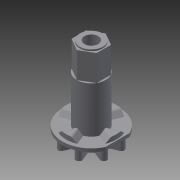
# Autodesk Inventor part: Picaporte
Saved by Autodesk Inventor 2014 (Build 180170000, 170)
## iProperties
Created: 2015-02-11
Part Number: Picaporte
Material: Generic
Document SubType Name: Modeling
Designer: Rubén
Density: 1 g/cm^3
Appearance: Default
Author: Rubén
Autodesk Inventor part; units mm, degrees
ref_plane "YZ Plane" through (0, 0, 0) normal (1, 0, 0) x (0, 1, 0)
ref_plane "XZ Plane" through (0, 0, 0) normal (0, 1, 0) x (-1, 0, 0)
ref_plane "XY Plane" through (0, 0, 0) normal (0, 0, 1) x (1, 0, 0)
sketch "Sketch1" plane through (0, 0, 0) normal (0, 1, 0) x (-1, 0, 0)
  arc A0 (-9.1, -4.1461) -> (-9.1, 4.1461) centre (0, 0) ccw
  line L0 (-9.1, 4.1461) -> (-9.1, -4.1461)
  dimension "d4" = 20
  dimension "d5" = 19.1
  constraints: 2 end point, 2 point on circle, 1 centre point, 1 coincident, 1 vertical
  measures "d4" diameter of A0
extrude "Extrusion1" add sketch "Sketch1" along normal blind 1.12
sketch "Sketch3" plane through (0, 1.12, 0) normal (0, 1, 0) x (1, 0, 0)
  arc A0 (9.1, 4.1461) -> (9.1, -4.1461) centre (0, 0) ccw projected
  circle A1 centre (0, 0) radius 5
  dimension "d14" = 10
  constraints: 1 centre point, 1 coincident
  measures "d14" diameter of A1
extrude "Extrusion3" add sketch "Sketch3" along normal blind 16
sketch "Sketch4" plane through (0, 17.12, 0) normal (0, 1, 0) x (1, 0, 0)
  circle A0 centre (0, 0) radius 5 projected
  line L0 (0, 5) -> (4.3301, 2.5)
  line L1 (4.3301, 2.5) -> (4.3301, -2.5)
  line L2 (4.3301, -2.5) -> (0, -5)
  line L3 (0, -5) -> (-4.3301, -2.5)
  line L4 (-4.3301, -2.5) -> (-4.3301, 2.5)
  line L5 (-4.3301, 2.5) -> (0, 5)
  constraints: 12 end point, 1 coincident, 1 vertical alignment, 14 other
extrude "Extrusion4" add sketch "Sketch4" along normal blind 9 contours L1 L2 L3 L4 L5 L0
sketch "Sketch5" plane through (0, 26.12, 0) normal (0, 1, 0) x (1, 0, 0)
  circle A0 centre (0, 0) radius 4
  dimension "d19" = 8
  constraints: 1 centre point, 1 coincident
  measures "d19" diameter of A0
extrude "Extrusion5" add sketch "Sketch5" along normal blind 0.5
sketch "Sketch6" plane through (0, 26.62, 0) normal (0, 1, 0) x (1, 0, 0)
  circle A0 centre (0, 0) radius 4 projected
hole "Hole1" at (0, 26.62, 0) direction (0, -1, 0) diameter 4.8 end through all
sketch "Sketch7" plane through (0, 1.12, 0) normal (0, 1, 0) x (1, 0, 0)
  circle A0 centre (0, 0) radius 5 projected
  arc A1 (9.1, 4.1461) -> (9.1, -4.1461) centre (0, 0) ccw projected
  arc A2 (3.25, 8.124) -> (-3.25, 8.124) centre (0, 0) ccw
  line L0 (0, 11.889) -> (0, 0) construction
  line L1 (-3.25, 8.124) -> (-1.8571, 4.6423)
  line L2 (3.25, 8.124) -> (1.8571, 4.6423)
  arc A3 (1.8571, 4.6423) -> (-1.8571, 4.6423) centre (0, 0) ccw
  arc A4 (-8.124, 3.25) -> (-8.124, -3.25) centre (0, 0) ccw
  line L3 (-8.124, -3.25) -> (-4.6423, -1.8571)
  line L4 (-8.124, 3.25) -> (-4.6423, 1.8571)
  arc A5 (-4.6423, 1.8571) -> (-4.6423, -1.8571) centre (0, 0) ccw
  arc A6 (-3.25, -8.124) -> (3.25, -8.124) centre (0, 0) ccw
  line L5 (3.25, -8.124) -> (1.8571, -4.6423)
  line L6 (-3.25, -8.124) -> (-1.8571, -4.6423)
  arc A7 (-1.8571, -4.6423) -> (1.8571, -4.6423) centre (0, 0) ccw
  arc A8 (8.124, -3.25) -> (8.124, 3.25) centre (0, 0) ccw
  line L7 (8.124, 3.25) -> (4.6423, 1.8571)
  line L8 (8.124, -3.25) -> (4.6423, -1.8571)
  arc A9 (4.6423, -1.8571) -> (4.6423, 1.8571) centre (0, 0) ccw
  dimension "d32" = 17.5
  dimension "d34" = 1.8571
  dimension "d35" = 3.25
  dimension "d36" = 4.6423
  dimension "d39" = 360
  constraints: 18 end point, 16 point on circle, 8 centre point, 2 symmetric about line, 1 coincident, 43 other
  measures "d32" diameter of A2
  measures "d34" distance from line of L0 L1.end
  measures "d35" distance from line of L0 L1.start
  measures "d36" vertical distance of point (0, 0) L1.end
extrude "Extrusion6" add sketch "Sketch7" along normal blind 1.6 contours A0 L7 A8 L8 | A0 L1 A2 L2 | L5 A6 L6 A0 | A0 L3 A4 L4
chamfer "Chamfer2" distance 1.6 angle 45 8 edges at (-2.5536, 2.72, -6.3832) (2.5536, 2.72, -6.3832) (-6.3832, 2.72, -2.5536) (-6.3832, 2.72, 2.5536) (-2.5536, 2.72, 6.3832) (2.5536, 2.72, 6.3832) (6.3832, 2.72, 2.5536) (6.3832, 2.72, -2.5536)
fillet "Fillet1" radius 1 8 edges at (6.7869, 2.72, -0.9919) (6.7869, 2.72, 0.9919) (0.9919, 2.72, 6.7869) (-0.9919, 2.72, 6.7869) (-6.7869, 2.72, 0.9919) (-6.7869, 2.72, -0.9919) (-0.9919, 2.72, -6.7869) (0.9919, 2.72, -6.7869)
sketch "Sketch8" plane through (0, 0, 0) normal (0, -1, 0) x (1, 0, 0)
  circle A0 centre (0, 0) radius 2.4 projected
  arc A1 (9.1, 4.1461) -> (9.1, -4.1461) centre (0, 0) ccw projected
  line L0 (0, 0) -> (9.2388, 3.8268) construction
  line L1 (0, 0) -> (10, 0) construction
  line L2 (3.9195, 2.7708) -> (6.9854, 4.0408)
  line L3 (8.292, 3.4996) -> (8.3149, 3.4442)
  arc A2 (8.292, 3.4996) -> (6.9854, 4.0408) centre (7.3681, 3.1169) ccw
  line L4 (4.7308, 0.8122) -> (7.7967, 2.0822)
  line L5 (8.3379, 3.3887) -> (8.3149, 3.4442)
  arc A3 (7.7967, 2.0822) -> (8.3379, 3.3887) centre (7.414, 3.006) ccw
  line L6 (0.8122, 4.7308) -> (2.0822, 7.7967)
  line L7 (3.3887, 8.3379) -> (3.4442, 8.3149)
  arc A4 (3.3887, 8.3379) -> (2.0822, 7.7967) centre (3.006, 7.414) ccw
  line L8 (2.7708, 3.9195) -> (4.0408, 6.9854)
  arc A5 (4.0408, 6.9854) -> (3.4996, 8.292) centre (3.1169, 7.3681) ccw
  line L9 (3.4996, 8.292) -> (3.4442, 8.3149)
  line L10 (-2.7708, 3.9195) -> (-4.0408, 6.9854)
  line L11 (-3.4996, 8.292) -> (-3.4442, 8.3149)
  arc A6 (-3.4996, 8.292) -> (-4.0408, 6.9854) centre (-3.1169, 7.3681) ccw
  line L12 (-0.8122, 4.7308) -> (-2.0822, 7.7967)
  arc A7 (-2.0822, 7.7967) -> (-3.3887, 8.3379) centre (-3.006, 7.414) ccw
  line L13 (-3.3887, 8.3379) -> (-3.4442, 8.3149)
  line L14 (-4.7308, 0.8122) -> (-7.7967, 2.0822)
  line L15 (-8.3379, 3.3887) -> (-8.3149, 3.4442)
  arc A8 (-8.3379, 3.3887) -> (-7.7967, 2.0822) centre (-7.414, 3.006) ccw
  line L16 (-3.9195, 2.7708) -> (-6.9854, 4.0408)
  arc A9 (-6.9854, 4.0408) -> (-8.292, 3.4996) centre (-7.3681, 3.1169) ccw
  line L17 (-8.292, 3.4996) -> (-8.3149, 3.4442)
  line L18 (-3.9195, -2.7708) -> (-6.9854, -4.0408)
  line L19 (-8.292, -3.4996) -> (-8.3149, -3.4442)
  arc A10 (-8.292, -3.4996) -> (-6.9854, -4.0408) centre (-7.3681, -3.1169) ccw
  line L20 (-4.7308, -0.8122) -> (-7.7967, -2.0822)
  arc A11 (-7.7967, -2.0822) -> (-8.3379, -3.3887) centre (-7.414, -3.006) ccw
  line L21 (-8.3379, -3.3887) -> (-8.3149, -3.4442)
  line L22 (-0.8122, -4.7308) -> (-2.0822, -7.7967)
  line L23 (-3.3887, -8.3379) -> (-3.4442, -8.3149)
  arc A12 (-3.3887, -8.3379) -> (-2.0822, -7.7967) centre (-3.006, -7.414) ccw
  line L24 (-2.7708, -3.9195) -> (-4.0408, -6.9854)
  arc A13 (-4.0408, -6.9854) -> (-3.4996, -8.292) centre (-3.1169, -7.3681) ccw
  line L25 (-3.4996, -8.292) -> (-3.4442, -8.3149)
  line L26 (2.7708, -3.9195) -> (4.0408, -6.9854)
  line L27 (3.4996, -8.292) -> (3.4442, -8.3149)
  arc A14 (3.4996, -8.292) -> (4.0408, -6.9854) centre (3.1169, -7.3681) ccw
  line L28 (0.8122, -4.7308) -> (2.0822, -7.7967)
  arc A15 (2.0822, -7.7967) -> (3.3887, -8.3379) centre (3.006, -7.414) ccw
  line L29 (3.3887, -8.3379) -> (3.4442, -8.3149)
  line L30 (4.7308, -0.8122) -> (7.7967, -2.0822)
  line L31 (8.3379, -3.3887) -> (8.3149, -3.4442)
  arc A16 (8.3379, -3.3887) -> (7.7967, -2.0822) centre (7.414, -3.006) ccw
  line L32 (3.9195, -2.7708) -> (6.9854, -4.0408)
  arc A17 (6.9854, -4.0408) -> (8.292, -3.4996) centre (7.3681, -3.1169) ccw
  line L33 (8.292, -3.4996) -> (8.3149, -3.4442)
  arc A18 (0.8122, 4.7308) -> (-0.8122, 4.7308) centre (0, 0) ccw
  arc A19 (-2.7708, 3.9195) -> (-3.9195, 2.7708) centre (0, 0) ccw
  arc A20 (-4.7308, 0.8122) -> (-4.7308, -0.8122) centre (0, 0) ccw
  arc A21 (-3.9195, -2.7708) -> (-2.7708, -3.9195) centre (0, 0) ccw
  arc A22 (-0.8122, -4.7308) -> (0.8122, -4.7308) centre (0, 0) ccw
  arc A23 (2.7708, -3.9195) -> (3.9195, -2.7708) centre (0, 0) ccw
  arc A24 (4.7308, -0.8122) -> (4.7308, 0.8122) centre (0, 0) ccw
  arc A25 (3.9195, 2.7708) -> (2.7708, 3.9195) centre (0, 0) ccw
  dimension "d50" = 22.5
  dimension "d51" = 1.06
  dimension "d52" = 9
  dimension "d53" = 1
  dimension "d56" = 360
  dimension "d58" = 4.8
  constraints: 68 end point, 49 point on circle, 24 centre point, 4 symmetric about line, 2 tangent, 1 coincident, 1 equal length, 1 horizontal, 1 parallel, 1 perpendicular, 1 point on line, 122 other
  measures "d50" angle of L1 L0
  measures "d51" distance between parallel lines of L0 L2
  measures "d52" distance from line of A0.centre L3
  measures "d53" radius of A2
  measures "d58" radius of A24
extrude "Extrusion7" add sketch "Sketch8" along normal blind 3.83
chamfer "Chamfer3" distance 2.2 angle 45 1 edges at (-2.4, -3.83, 0)
body "Solid1"
